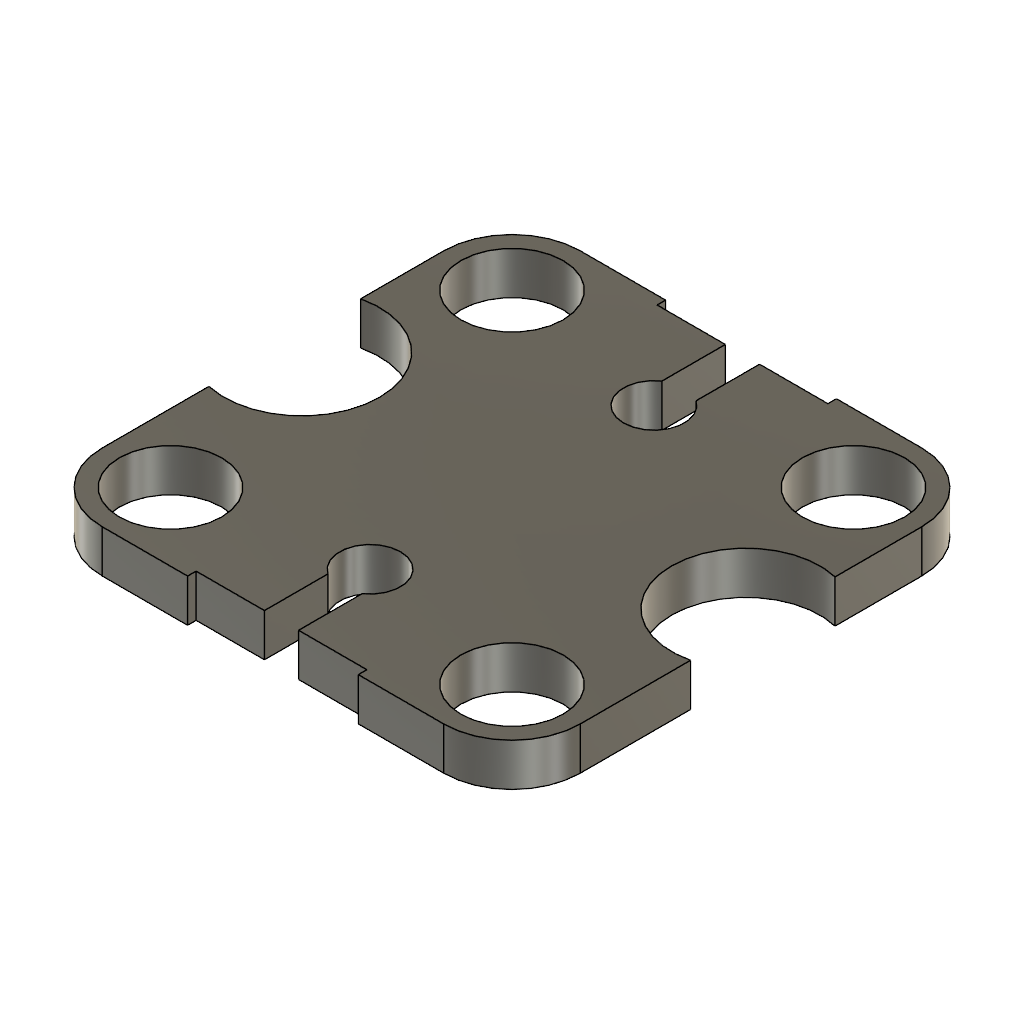
exercise 15 (Autodesk Fusion 360 design; units mm, degrees)
part number: 2026-10-09-21-48-19-307
Autodesk Fusion 360 part; units mm, degrees
sketch "Sketch1" plane through (0, 0, 0) normal (0, 0, 1) x (1, 0, 0)
  circle A0 centre (-55.475, -25) radius 30
  circle A1 centre (144.525, -25) radius 30
  circle A2 centre (144.525, -225) radius 30
  circle A3 centre (-55.475, -225) radius 30
  line L0 (-55.475, 15) -> (144.525, 15)
  line L1 (144.525, -265) -> (-55.475, -265)
  line L2 (-95.475, 15) -> (184.525, -265) construction
  line L3 (184.525, 15) -> (-95.475, -265) construction
  line L4 (184.525, -25) -> (184.525, -75.8302)
  line L5 (184.525, -160.367) -> (184.525, -225)
  arc A4 (184.525, -75.8302) -> (184.525, -160.367) centre (174.525, -118.0986) ccw
  line L6 (-95.475, -225) -> (-95.475, -162.4976)
  line L7 (-95.475, -73.6997) -> (-95.475, -25)
  arc A5 (-95.475, -162.4976) -> (-95.475, -73.6997) centre (-85.475, -118.0986) ccw
  arc A6 (-55.475, 15) -> (-95.475, -25) centre (-55.475, -25) ccw
  arc A7 (184.525, -25) -> (144.525, 15) centre (144.525, -25) ccw
  arc A8 (144.525, -265) -> (184.525, -225) centre (144.525, -225) ccw
  arc A9 (-95.475, -225) -> (-55.475, -265) centre (-55.475, -225) ccw
  line L8 (-5.475, -265) -> (-5.475, -260)
  line L9 (94.525, -265) -> (94.525, -260)
  line L10 (-5.475, -260) -> (34.525, -260)
  line L11 (94.525, -260) -> (54.525, -260)
  line L12 (34.525, -260) -> (34.525, -222.8224)
  line L13 (54.525, -260) -> (54.525, -222.8224)
  arc A10 (54.525, -222.8224) -> (34.525, -222.8224) centre (44.525, -208.0986) ccw
  line L14 (34.525, 10) -> (34.525, -27.1776)
  arc A11 (34.525, -27.1776) -> (54.525, -27.1776) centre (44.525, -41.9014) ccw
  line L15 (54.525, 10) -> (54.525, -27.1776)
  line L16 (-5.475, 10) -> (34.525, 10)
  line L17 (94.525, 10) -> (54.525, 10)
  line L18 (-5.475, 15) -> (-5.475, 10)
  line L19 (94.525, 15) -> (94.525, 10)
  point P0 (44.525, -125)
  dimension "d1" = 60
  dimension "d2" = 60
  dimension "d3" = 200
  dimension "d4" = 200
  dimension "d5" = 200
  dimension "d8" = 260
  dimension "d9" = 280
  dimension "d10" = 280
  dimension "d11" = 40
  dimension "d12" = 40
  dimension "d13" = 40
  dimension "d14" = 40
  dimension "d15" = 40
  dimension "d16" = 40
  dimension "d17" = 40
  dimension "d18" = 100
  dimension "d19" = 50
  dimension "d20" = 5
  dimension "d21" = 5
  dimension "d22" = 40
  dimension "d23" = 40
  constraint horizontal L0
  constraint perpendicular L0 L4
  constraint parallel L0 L1
  constraint parallel L4 L7
  constraint coincident L2 P0
  constraint coincident L3 P0
  constraint collinear L4 L5
  constraint collinear L6 L7
  constraint coincident L2.start L7
  constraint coincident L2.start L0
  constraint tangent L7 A6
  constraint tangent L0 A6
  constraint coincident L3.start L0
  constraint coincident L3.start L4
  constraint tangent L0 A7
  constraint tangent L4 A7
  constraint coincident L2.end L1
  constraint coincident L2.end L5
  constraint tangent L1 A8
  constraint tangent L5 A8
  constraint coincident L3.end L6
  constraint coincident L3.end L1
  constraint tangent L6 A9
  constraint tangent L1 A9
  constraint coincident L1 L8.start
  constraint perpendicular L1 L9
  constraint perpendicular L8 L10
  constraint perpendicular L9 L11
  constraint perpendicular L10 L12
  constraint perpendicular L11 L13
  measures "d1" diameter of A0
  measures "d2" diameter of A1
  measures "d3" horizontal distance of A0.centre A1.centre
  measures "d4" distance of A0.centre A3.centre
  measures "d5" distance of A1.centre A2.centre
  measures "d8" distance of A5.centre A4.centre
  measures "d9" distance of L2.end L3.end
  measures "d10" distance of L3.start L2.end
  measures "d11" distance of A0.centre L0
  measures "d12" distance of A1.centre L0
  measures "d13" distance of A1.centre L4
  measures "d14" radius of A6
  measures "d15" radius of A7
  measures "d16" radius of A8
  measures "d17" radius of A9
  measures "d18" distance of L8.start L9.start
  measures "d19" horizontal distance of A3.centre L8.start
  measures "d20" distance of L8.start L8.end
  measures "d21" distance of L9.start L9.end
  measures "d22" distance of L8.end L10.end
  measures "d23" distance of L9.end L11.end
extrude "Extrude1" add sketch "Sketch1" along normal blind 25 contours L0 L1 L4 L5 A4 L6 L7 A5 A6 A7 A8 A9 L8 L9 L10 L11 L12 L13 A10 L14 A11 L15 L16 L17 L18 L19
